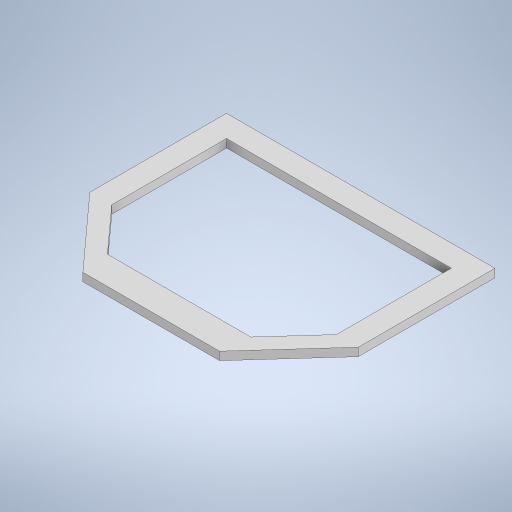
# Autodesk Inventor part: TopServoMount02
Saved by Autodesk Inventor 2024.2 (Build 282272000, 272)
## iProperties
Created: 2024-04-02
Part Number: TopServoMount02
Material: Generic
Document SubType Name: Modeling
Designer: ringl
Density: 1 g/cm^3
Appearance: Default
Author: ringl
Autodesk Inventor part; units mm, degrees
ref_plane "YZ Plane" through (0, 0, 0) normal (1, 0, 0) x (0, 1, 0)
ref_plane "XZ Plane" through (0, 0, 0) normal (0, 1, 0) x (-1, 0, 0)
ref_plane "XY Plane" through (0, 0, 0) normal (0, 0, 1) x (1, 0, 0)
sketch "Sketch1" plane through (0, 0, 0) normal (0, 1, 0) x (-1, 0, 0)
  line L0 (98.2, 0) -> (98.2, -50)
  line L1 (0, -50) -> (0, 0)
  line L2 (24.1, 26.635) -> (74.1, 26.635)
  line L3 (24.1, 26.635) -> (0, 0)
  line L4 (74.1, 26.635) -> (98.2, 0)
  line L5 (8, 0) -> (8, -42)
  line L6 (90.2, -42) -> (90.2, 0)
  line L7 (90.2, 0) -> (75.3278, 16.4366)
  line L8 (75.3278, 16.4366) -> (22.8722, 16.4366)
  line L9 (22.8722, 16.4366) -> (8, 0)
  line L10 (90.2, -42) -> (8, -42)
  line L11 (98.2, -50) -> (0, -50)
  dimension "d0" = 98.2
  dimension "d1" = 50
  dimension "d2" = 50
  dimension "d5" = 26.635
  dimension "d6" = 24.1
  dimension "d7" = 24.1
  dimension "d9" = 8
  dimension "d10" = 8
  dimension "d11" = 42
  constraints: 24 end point, 3 horizontal alignment, 3 parallel, 2 horizontal, 1 perpendicular, 1 vertical, 1 vertical alignment
  measures "d0" distance of L0.end L1.start
  measures "d1" distance of L1.start L1.end
  measures "d2" distance of L2.start L2.end
  measures "d5" distance from line of L1.end L2
  measures "d6" horizontal distance of L1.end L2.start
  measures "d7" horizontal distance of L0.start L2.end
  measures "d9" distance between parallel lines of L0 L6
  measures "d10" distance between parallel lines of L1 L5
  measures "d11" distance of L6.start L6.end
extrude "Extrusion1" add sketch "Sketch1" along normal blind 3
body "Solid1"
